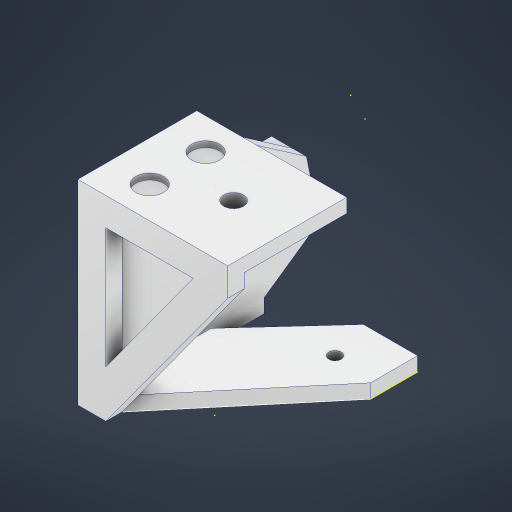
# Autodesk Inventor part: DC23[R][F][T1]
Saved by Autodesk Inventor 2024 (Build 280153000, 153)
## iProperties
Created: 2022-10-25
Part Number: DC23[R][F][T1]
Material: Aluminio 6061
Document SubType Name: Modeling
Designer: juanr
Density: 2.7 g/cm^3
Appearance: Aluminio - Plano
Mass: 248.976 g
Surface Area: 332.545 cm^2
Volume: 92.2132 cm^3
Author: juanr
Autodesk Inventor part; units mm, degrees
ref_plane "YZ Plane" through (0, 0, 0) normal (1, 0, 0) x (0, 1, 0)
ref_plane "XZ Plane" through (0, 0, 0) normal (0, 1, 0) x (-1, 0, 0)
ref_plane "XY Plane" through (0, 0, 0) normal (0, 0, 1) x (1, 0, 0)
sketch "Sketch1" plane through (0, 0, 0) normal (0, 1, 0) x (-1, 0, 0)
  line L0 (0, -25.5) -> (-34.15, -25.5)
  line L1 (-34.15, -25.5) -> (-34.15, 0)
  line L2 (-34.15, 0) -> (-34.15, 25.5)
  line L3 (-34.15, 25.5) -> (0, 25.5)
  line L4 (0, 25.5) -> (34.15, 25.5)
  line L5 (34.15, 25.5) -> (34.15, 0)
  line L6 (34.15, 0) -> (34.15, -25.5)
  line L7 (34.15, -25.5) -> (0, -25.5)
  point P0 (0, 0)
  constraints: 16 end point, 3 perpendicular, 2 point on line, 1 horizontal, 1 vertical
extrude "Extrusion1" add sketch "Sketch1" along normal blind 7
sketch "Sketch3" plane through (-34.15, 0, 25.5) normal (0, 0, 1) x (1, 0, 0)
  line L0 (0, 0) -> (0, -78.85)
  point P0 (34.15, 0)
  dimension "d7" = 78.85
  constraints: 2 end point, 1 vertical
  measures "d7" distance of L0.start L0.end
sketch "Sketch4" plane through (-34.15, 0, -25.5) normal (-1, 0, 0) x (0, 0, 1)
  line L0 (51, 0) -> (51, -78.85)
  line L1 (51, -78.85) -> (-39, -78.85)
  line L2 (-39, -78.85) -> (-39, -71.85)
  line L3 (0, 0) -> (-39, -71.85)
  line L4 (0, 0) -> (51, 0)
  point P0 (25.5, 0)
  dimension "d10" = 90
  dimension "d11" = 7
  constraints: 10 end point, 2 horizontal, 2 vertical
  measures "d10" distance of L0.end L1.end
  measures "d11" distance of L1.end L2.end
extrude "Extrusion2" add sketch "Sketch4" against normal blind 7
sketch "Sketch6" plane through (0, 7, 0) normal (0, 1, 0) x (1, 0, 0)
  line L0 (34.15, -25.5) -> (34.15, 25.5) projected
  line L1 (34.15, 25.5) -> (34.15, 0)
  line L2 (-34.15, 25.5) -> (-34.15, -25.5) projected
  circle A0 centre (8.15, 0) radius 5
  point P0 (0, 0)
  dimension "d20" = 10
  constraints: 2 end point, 1 centre point, 1 midpoint
  measures "d20" diameter of A0
extrude "Extrusion4" cut sketch "Sketch6" against normal blind 10
sketch "Sketch7" plane through (-27.15, 0, -25.5) normal (1, 0, 0) x (0, 0, -1)
  line L0 (-51, -78.85) -> (39, -78.85) projected
  line L1 (-51, -78.85) -> (39, -78.85)
  line L2 (39, -78.85) -> (39, -71.85) projected
  line L3 (39, -78.85) -> (39, -71.85)
  line L4 (39, -71.85) -> (-51, -71.85)
  line L5 (-51, 0) -> (-51, -78.85) projected
  line L6 (-51, -78.85) -> (-51, -71.85)
  point P0 (-25.5, 0)
  constraints: 8 end point, 2 perpendicular, 1 collinear, 1 horizontal, 1 point on line
sketch "Sketch8" plane through (0, 0, 0) normal (0, -1, 0) x (1, 0, 0)
  circle A0 centre (8.15, 0) radius 5 projected
  line L0 (8.15, 18.5) -> (34.15, 18.5)
  line L1 (34.15, 25.5) -> (34.15, -25.5) projected
  line L2 (8.15, 25.5) -> (34.15, 25.5)
  line L3 (8.15, 25.5) -> (-27.15, 25.5)
  line L4 (-27.15, 25.5) -> (-27.15, -25.5) projected
  line L5 (8.15, 18.5) -> (-27.15, 18.5)
  line L6 (34.15, 25.5) -> (34.15, 18.5)
  line L7 (-27.15, 25.5) -> (-27.15, 18.5)
  point P0 (0, 0)
  constraints: 12 end point, 2 collinear, 2 point on line, 1 horizontal, 1 parallel
extrude "Extrusion6" add sketch "Sketch7" along normal blind 58.5
extrude "Extrusion7" add sketch "Sketch8" along normal blind 78.75 contours L5 L4 L3 L2 L1 L0
sketch "Sketch9" plane through (31.35, 0, -25.5) normal (1, 0, 0) x (0, 0, -1)
  line L0 (-51, -78.75) -> (-51, 7) projected
  line L1 (-44, 0) -> (-44, -71.85) projected
  line L2 (-51, -78.75) -> (-44, -78.75)
  line L3 (-44, -78.75) -> (-44, -71.85)
  line L4 (-44, -71.85) -> (-51, -71.85)
  line L5 (-51, -71.85) -> (-51, -78.75)
  point P0 (-25.5, 0)
  constraints: 8 end point, 2 parallel, 1 horizontal, 1 perpendicular
extrude "Extrusion8" cut sketch "Sketch9" along normal blind 10
sketch "Sketch10" plane through (0, 7, 0) normal (0, 1, 0) x (1, 0, 0)
  point P0 (0, 0)
sketch "Boceto11" plane through (-34.15, -78.85, -64.5) normal (0, -1, 0) x (1, 0, 0)
  line L0 (72.0718, 89.9914) -> (72.0718, 37.9883)
  line L1 (72.0718, 37.9883) -> (65.5278, 37.9883)
  line L2 (65.5278, 37.9883) -> (65.5278, 89.9914)
  line L3 (72.0718, 89.9914) -> (72.0718, 92.1751)
  line L4 (72.0718, 92.1751) -> (65.5278, 92.1751)
  line L5 (65.5278, 92.1751) -> (65.5278, 89.9914)
  point P0 (34.15, 64.5)
  constraints: 12 end point, 2 perpendicular, 1 parallel, 1 vertical
extrude "Extrusión9" cut sketch "Boceto11" against normal blind 1000
sketch "Boceto18" plane through (-34.15, -78.85, 25.5) normal (0, 0, 1) x (1, 0, 0)
  point P0 (34.15, 78.85)
sketch "Boceto23" plane through (-27.15, 0, -25.5) normal (0, 0.4770514, -0.8788754) x (-1, 0, 0)
  point P0 (-27.15, 12.1648)
sketch "Boceto24" plane through (-27.15, 0, -25.5) normal (0, 0, -1) x (-1, 0, 0)
  line L0 (7, -71.85) -> (7, -78.85) projected
  line L1 (7, -78.35) -> (7, -78.85)
  line L2 (7, -78.85) -> (-58.5, -78.85) projected
  line L3 (-58.5, -78.85) -> (-58.5, -77.85)
  line L4 (-58.5, -71.85) -> (-58.5, -78.85) projected
  line L5 (-58.5, -77.85) -> (6, -77.85)
  line L6 (7, -77.85) -> (7, -78.85)
  line L7 (7, -78.85) -> (-58.8392, -78.85)
  line L8 (-58.5278, 7) -> (7, 7) projected
  line L9 (7, -78.85) -> (7, 7)
  line L10 (7, 7) -> (6, 7)
  line L11 (6, 6) -> (6, -77.85)
  line L12 (-58.5278, -71.85) -> (-58.5278, 7) projected
  line L13 (-58.5278, 7) -> (-58.5278, 6)
  line L14 (-58.5278, 6) -> (6, 6)
  line L15 (7, 0) -> (7, 7) projected
  line L16 (7, 6) -> (7, 7)
  line L17 (7, 7) -> (-58.5278, 7)
  point P0 (-27.15, 0)
  dimension "d65" = 1
  dimension "d66" = 1
  dimension "d67" = 1
  constraints: 24 end point, 7 perpendicular, 5 point on line, 1 collinear, 1 horizontal, 1 vertical
  measures "d65" distance of L2.end L3.end
  measures "d66" distance of L8.end L10.end
  measures "d67" distance of L8.start L13.end
extrude "Extrusión19" cut sketch "Boceto24" along normal mid plane 1000
sketch "Boceto25" plane through (31.35, -71.85, -64.5) normal (0, 0, -1) x (-1, 0, 0)
  point P0 (31.35, 71.85)
sketch "Boceto27" plane through (31.3778, 0, -25.5) normal (0, 0, -1) x (-1, 0, 0)
  line L0 (0, -71.85) -> (0, 6) projected
  line L1 (0, 6) -> (0.228, 6)
  line L2 (0, 6) -> (64.5278, 6) projected
  line L3 (0.228, 6) -> (0.228, -77.85)
  line L4 (0.0278, -77.85) -> (64.5278, -77.85) projected
  line L5 (0.0278, -71.85) -> (0.0278, -77.85) projected
  line L6 (0.228, -77.85) -> (0.0278, -77.85)
  line L7 (0.0278, -77.85) -> (0, 6)
  line L8 (0, 6) -> (0, -77.85)
  line L9 (0, -77.85) -> (0.0278, -77.85)
  point P0 (31.3778, 0)
  dimension "d73" = 0.228
  constraints: 12 end point, 3 perpendicular, 3 point on line, 1 horizontal
  measures "d73" distance of L0.end L1.end
extrude "Extrusión21" cut sketch "Boceto27" along normal mid plane 1000
sketch "Boceto28" plane through (-33.15, 0, -25.5) normal (-1, 0, 0) x (0, 0, 1)
  point P0 (25.5, 0)
sketch "Boceto30" plane through (-33.15, 0, -25.5) normal (-1, 0, 0) x (0, 0, 1)
  point P0 (25.5, 0)
sketch "Boceto31" plane through (-33.15, 0, -25.5) normal (-1, 0, 0) x (0, 0, 1)
  circle A0 centre (64.38, -38.5153) radius 2.6
  point P0 (25.5, 0)
  point P1 (64.38, -49.4573)
  constraints: 1 centre point
sketch "Boceto32" plane through (-27.15, -71.85, 18.5) normal (0, 1, 0) x (1, 0, 0)
  circle A0 centre (47, 71.5) radius 5 projected
  circle A1 centre (47, 71.5) radius 5
  line L0 (52, 71.5) -> (58.2998, 71.5)
  line L1 (67, 83) -> (67, -7)
  line L2 (58.2998, -7) -> (-6, -7) projected
  line L3 (67, -7) -> (58.2998, -7)
  line L4 (58.2998, -7) -> (58.2998, 83)
  line L5 (47, 76.5) -> (47, 83)
  line L6 (-6, 83) -> (0, 83) projected
  line L7 (-6, 83) -> (-6, 91.5)
  line L8 (-6, 91.5) -> (67, 91.5)
  line L9 (67, 91.5) -> (67, 83)
  line L10 (-6, 83) -> (58.2998, 83)
  point P0 (27.15, 18.5)
  constraints: 18 end point, 2 perpendicular, 2 point on circle, 2 point on line, 2 vertical, 1 centre point, 1 coincident, 1 collinear, 1 horizontal
extrude "Extrusión23" add sketch "Boceto32" against normal blind 6 contours L4 L10 L6 L7 L8 L9 L1 L3
sketch "Boceto33" plane through (-33.15, -77.85, 25.5) normal (-1, 0, 0) x (0, 0, 1)
  line L0 (0, 83.85) -> (0, 0) projected
  line L1 (0, 74.4354) -> (10.1255, 74.4354)
  line L2 (10.1255, 74.4354) -> (10.1255, 56.6115)
  line L3 (10.9445, 54.9975) -> (18.0243, 49.8171)
  line L4 (18.8039, 48.5979) -> (20.1084, 42.1205)
  line L5 (0, 11.6181) -> (18.1478, 11.6181)
  line L6 (20.1478, 13.6181) -> (20.1478, 41.7256)
  arc A0 (10.1255, 56.6115) -> (10.9445, 54.9975) centre (12.1255, 56.6115) ccw
  arc A1 (18.8039, 48.5979) -> (18.0243, 49.8171) centre (16.8433, 48.203) ccw
  arc A2 (20.1478, 41.7256) -> (20.1084, 42.1205) centre (18.1478, 41.7256) ccw
  arc A3 (18.1478, 11.6181) -> (20.1478, 13.6181) centre (18.1478, 13.6181) ccw
  point P0 (-25.5, 77.85)
  dimension "d91" = 2
  constraints: 12 end point, 8 point on circle, 8 tangent, 4 centre point, 3 equal radius, 2 horizontal, 2 perpendicular, 2 point on line
  measures "d91" radius of A0
extrude "Extrusión24" add sketch "Boceto33" against normal blind 6
extrude "Extrusión25" cut sketch "Boceto31" against normal blind 6
sketch "Boceto34" plane through (-27.15, -77.85, 25.5) normal (1, 0, 0) x (0, 0, -1)
  line L0 (-18.1478, 11.6181) -> (-21.8775, 11.6181)
  line L1 (-21.8775, 11.6181) -> (-21.8775, 48.067)
  line L2 (-21.8775, 48.067) -> (-10.1255, 56.8358)
  line L3 (-10.1255, 74.4354) -> (-10.1255, 56.6115) projected
  line L4 (-10.1255, 56.8358) -> (-10.1255, 48.9642)
  line L5 (-10.1255, 48.9642) -> (-16.6729, 42.1735)
  line L6 (-16.6729, 42.1735) -> (-18.1478, 11.6181)
  point P0 (25.5, 77.85)
  constraints: 12 end point, 1 horizontal, 1 perpendicular, 1 point on line, 1 vertical
extrude "Extrusión26" add sketch "Boceto34" against normal blind 6
fillet "Empalme5" radius 10 3 edges at (-30.15, -21.0142, 35.6255) (-30.15, -29.783, 47.3775) (-30.15, -66.2319, 47.3775)
sketch "Boceto37" plane through (-33.15, 6, 25.5) normal (0, 1, 0) x (1, 0, 0)
  circle A0 centre (41.3, 25.5) radius 6 projected
  line L0 (41.3, 25.5) -> (17.3, 25.5)
  line L1 (17.3, 25.5) -> (17.3, 13.5)
  line L2 (17.3, 13.5) -> (17.3, 37.5)
  circle A1 centre (17.3, 13.5) radius 6
  circle A2 centre (17.3, 37.5) radius 6
  point P0 (33.15, 25.5)
  dimension "d106" = 24
  dimension "d107" = 12
  dimension "d108" = 24
  dimension "d109" = 12
  dimension "d110" = 12
  constraints: 6 end point, 2 centre point, 2 coincident, 1 horizontal, 1 perpendicular, 1 point on line
  measures "d106" distance of L0.start L0.end
  measures "d107" distance of L0.end L1.end
  measures "d108" distance of L1.end L2.end
  measures "d109" diameter of A1
  measures "d110" diameter of A2
extrude "Extrusión29" cut sketch "Boceto37" against normal blind 2.5 contours A1 | A2
sketch "Boceto39" plane through (-27.15, -71.85, 18.5) normal (0, 1, 0) x (1, 0, 0)
  line L0 (58.2998, -7) -> (58.2998, 0)
  line L1 (58.2998, 44) -> (58.2998, 91.5)
  line L2 (-6, 91.5) -> (67, 91.5) projected
  line L3 (0, 0) -> (58.2998, 0) projected
  line L4 (58.2998, 0) -> (58.2998, -7) projected
  line L5 (58.2998, -7) -> (67, -7) projected
  line L6 (58.2998, -7) -> (67, -7)
  line L7 (67, 91.5) -> (-6, 91.5) projected
  line L8 (67, -7) -> (67, 91.5)
  line L9 (67, 91.5) -> (58.2998, 91.5)
  line L10 (58.2998, 0) -> (58.2998, 44)
  point P0 (27.15, 18.5)
  constraints: 12 end point, 3 collinear, 2 point on line, 1 perpendicular, 1 vertical
extrude "Extrusión31" cut sketch "Boceto39" against normal blind 10
sketch "Boceto41" plane through (-27.15, -71.85, 18.5) normal (0, 1, 0) x (1, 0, 0)
  line L0 (58.2998, 91.5) -> (58.2998, -7) projected
  line L1 (58.2998, 91.5) -> (31.7998, 91.5)
  line L2 (31.7998, 91.5) -> (31.7998, 65)
  line L3 (31.7998, 65) -> (58.2998, 65)
  line L4 (58.2998, 65) -> (58.2998, 91.5)
  circle A0 centre (31.7998, 65) radius 6
  point P0 (27.15, 18.5)
  dimension "d124" = 26.5
  dimension "d125" = 26.5
  dimension "d126" = 12
  constraints: 8 end point, 2 parallel, 1 centre point, 1 coincident, 1 horizontal, 1 perpendicular
  measures "d124" distance of L3.end L2.end
  measures "d125" distance of L2.end L1.end
  measures "d126" diameter of A0
extrude "Extrusión32" cut sketch "Boceto41" against normal blind 10 contours A0 L2 L3 | L3 L2 A0
sketch "Sketch42" plane through (-27.15, -71.85, 18.5) normal (0, 1, 0) x (1, 0, 0)
  circle A0 centre (31.7998, 65) radius 6 projected
  line L0 (31.7998, 71) -> (31.7998, 65)
  circle A1 centre (31.7998, 65) radius 18
  line L1 (0, 0) -> (0, 83) projected
  line L2 (0, 83) -> (31.7998, 83)
  line L3 (58.2998, 91.5) -> (-6, 91.5) projected
  line L4 (49.7998, 65) -> (49.7998, 0)
  line L5 (58.2998, 0) -> (0, 0) projected
  line L6 (0, 0) -> (58.2998, 0) projected
  line L7 (49.7998, 0) -> (58.2998, 0)
  line L8 (58.2998, 91.5) -> (58.2998, -7) projected
  line L9 (58.2998, 0) -> (58.2998, 91.5)
  line L10 (0, 83) -> (0, 44) projected
  line L11 (0, 83) -> (-6, 83)
  line L12 (-6, 91.5) -> (-6, 83) projected
  line L13 (-6, 83) -> (-6, 91.5)
  line L14 (58.2998, 91.5) -> (58.2998, 0) projected
  line L15 (-6, 91.5) -> (58.2998, 91.5)
  point P0 (27.15, 18.5)
  point P1 (58.2998, -7)
  dimension "d129" = 36
  constraints: 16 end point, 3 vertical, 2 collinear, 2 point on circle, 1 centre point, 1 coincident, 1 horizontal, 1 parallel, 1 perpendicular, 1 point on line, 1 vertical alignment, 2 other
  measures "d129" diameter of A1
extrude "Extrusion33" cut sketch "Sketch42" against normal blind 10 contours A1 L2 L11 L12 L3 L8 L5 L4
sketch "Sketch43" plane through (-27.15, -71.85, 18.5) normal (0, 0, -1) x (-1, 0, 0)
  line L0 (6, -6) -> (-58.2998, -6) projected
  line L1 (0, 0) -> (-49.7998, 0) projected
  line L2 (-58.2998, -6) -> (-49.7998, -6)
  line L3 (-49.7998, -6) -> (-49.7998, 0)
  line L4 (-49.7998, 0) -> (-58.2998, 0)
  line L5 (-58.2998, 0) -> (-58.2998, -6)
  point P0 (-27.15, 71.85)
  constraints: 8 end point, 2 parallel, 1 horizontal, 1 perpendicular
extrude "Extrusion34" add sketch "Sketch43" along normal blind 20
fillet "Fillet7" radius 7 1 edges at (31.1498, -74.85, -1.5)
fillet "Fillet8" radius 2 1 edges at (22.6498, -74.85, -1.5)
sketch "Sketch44" plane through (-33.15, 0, -25.5) normal (-1, 0, 0) x (0, 0, 1)
  line L0 (68.8577, -26.7837) -> (65.1452, -24.0136) projected
  line L1 (61.1255, -3.4146) -> (51, -3.4146) projected
  line L2 (65.1452, -24.0136) -> (51, -24.0136)
  line L3 (51, -24.0136) -> (51, -3.4146)
  line L4 (51, -3.4146) -> (65.1452, -3.4146)
  line L5 (65.1452, -3.4146) -> (65.1452, -24.0136)
  point P0 (25.5, 0)
  constraints: 8 end point, 2 parallel, 1 horizontal, 1 perpendicular
extrude "Extrusion35" cut sketch "Sketch44" against normal blind 20
sketch "Sketch45" plane through (-33.15, 6, 25.5) normal (0, 1, 0) x (1, 0, 0)
  circle A0 centre (41.3, 25.5) radius 5 projected
  circle A1 centre (41.3, 25.5) radius 4.25
  circle A2 centre (41.3, 25.5) radius 5
  point P0 (33.15, 25.5)
  dimension "d138" = 8.5
  constraints: 2 centre point, 2 coincident, 1 concentric
  measures "d138" diameter of A1
extrude "Extrusion36" add sketch "Sketch45" against normal blind 6
sketch "Sketch46" plane through (-33.15, 0, -25.5) normal (-1, 0, 0) x (0, 0, 1)
  point P0 (25.5, 0)
sketch "Sketch47" plane through (-33.15, 0, -25.5) normal (-1, 0, 0) x (0, 0, 1)
  line L0 (-44.1201, -43.7798) -> (-41.0263, -28.4947)
  line L1 (-39, -71.85) -> (0, 0) projected
  line L2 (-41.0263, -28.4947) -> (0, 0)
  line L3 (0, 0) -> (-39, -71.85)
  line L4 (-44.1201, -43.7798) -> (-44.1201, -71.85)
  line L5 (-44.1201, -71.85) -> (-39, -71.85)
  point P0 (25.5, 0)
  constraints: 10 end point, 1 collinear, 1 perpendicular, 1 vertical
extrude "Extrusion37" add sketch "Sketch47" against normal blind 6
sketch "Sketch48" plane through (-33.15, 6, -25.5) normal (-1, 0, 0) x (0, 0, 1)
  point P0 (25.5, -6)
sketch "Sketch49" plane through (-33.15, 6, -25.5) normal (-1, 0, 0) x (0, 0, 1)
  point P0 (25.5, -6)
sketch "Sketch50" plane through (-33.15, 6, -25.5) normal (-1, 0, 0) x (0, 0, 1)
  line L0 (-44.1201, -49.7798) -> (-41.0263, -34.4947) projected
  line L1 (-41.0263, -34.4947) -> (-46.4891, -61.4839)
  line L2 (-39, -83.85) -> (51, -83.85) projected
  line L3 (-39, -83.85) -> (-46.4891, -83.85)
  line L4 (-46.4891, -83.85) -> (-46.4891, -61.4839)
  line L5 (-41.0263, -34.4947) -> (-39, -69.2782)
  line L6 (-39, -69.2782) -> (-39, -83.85)
  point P0 (25.5, -6)
  constraints: 10 end point, 1 collinear, 1 horizontal, 1 perpendicular, 1 vertical
extrude "Extrusion38" add sketch "Sketch50" against normal blind 6
sketch "Sketch51" plane through (-33.15, 6, -25.5) normal (-1, 0, 0) x (0, 0, 1)
  line L0 (-41.0263, -34.4947) -> (-46.4891, -61.4839) projected
  line L1 (-41.0263, -34.4947) -> (-46.4891, -61.4839)
  line L2 (-46.4891, -61.4839) -> (-15.8808, -61.4839)
  line L3 (-41.0263, -34.4947) -> (-15.8808, -34.4947)
  line L4 (-15.8808, -34.4947) -> (-15.8808, -61.4839)
  point P0 (25.5, -6)
  constraints: 8 end point, 2 horizontal, 1 collinear, 1 perpendicular
extrude "Extrusion39" add sketch "Sketch51" along normal blind 9
sketch "Sketch52" plane through (-33.15, -55.4839, -71.9891) normal (0, -1, 0) x (1, 0, 0)
  line L0 (-9, 30.6084) -> (0, 53.8004)
  line L1 (0, 0) -> (0, 97.4891) projected
  line L2 (0, 30.6084) -> (0, 53.8004)
  line L3 (0, 30.6084) -> (-9, 30.6084)
  point P0 (33.15, 71.9891)
  constraints: 6 end point, 2 point on line, 1 collinear, 1 perpendicular
extrude "Extrusion40" add sketch "Sketch52" against normal blind 26.989
sketch "Sketch53" plane through (-33.15, -55.4839, -18.1887) normal (-0.9322642, 0, 0.3617781) x (0.3617781, 0, 0.9322642)
  point P0 (28.9496, 55.4839)
sketch "Sketch54" plane through (-33.15, 6, -25.5) normal (-1, 0, 0) x (0, 0, 1)
  line L0 (51, -72.2319) -> (51, -83.85) projected
  line L1 (51, -83.85) -> (86.3988, -83.85)
  line L2 (86.3988, -83.85) -> (86.3988, -18.2813)
  line L3 (86.3988, -18.2813) -> (51, -18.2813)
  line L4 (51, -18.2813) -> (51, -83.85)
  point P0 (25.5, -6)
  constraints: 8 end point, 2 parallel, 1 horizontal, 1 perpendicular
extrude "Extrusion41" cut sketch "Sketch54" against normal blind 26.989
sketch "Sketch55" plane through (-33.15, -55.4839, -71.9891) normal (0, 0.198384, -0.9801244) x (-1, 0, 0)
  line L0 (9, 6.0722) -> (9, 32.5248) projected
  line L1 (9, 17.5562) -> (3.5, 17.5562)
  line L2 (9, 17.5562) -> (14.5, 17.5562) construction
  circle A0 centre (3.5, 17.5562) radius 2.55
  point P0 (-33.15, 68.6627)
  dimension "d153" = 5.5
  dimension "d154" = 180
  dimension "d155" = 5.1
  constraints: 4 end point, 1 centre point, 1 coincident, 1 collinear, 1 horizontal, 1 perpendicular, 1 point on line
  measures "d153" distance of L1.start L1.end
  measures "d154" angle of L1 L2
  measures "d155" diameter of A0
extrude "Extrusion42" cut sketch "Sketch55" against normal blind 20
sketch "Sketch56" plane through (-33.15, -77.85, 25.5) normal (0, 0, 1) x (1, 0, 0)
  line L0 (0, 77.85) -> (0, 83.85) projected
  line L1 (0, 83.85) -> (12, 83.85)
  line L2 (64.2998, 83.85) -> (0, 83.85) projected
  line L3 (12, 83.85) -> (12, 0)
  line L4 (6, 0) -> (37.7998, 0) projected
  line L5 (0, 83.85) -> (0, 0) projected
  line L6 (12, 0) -> (0, 0)
  line L7 (0, 0) -> (0, 83.85)
  line L8 (0, 83.85) -> (12, 83.85)
  line L9 (12, 83.85) -> (12, 0)
  line L10 (0, 83.85) -> (64.3, 83.85)
  line L11 (64.3, 83.85) -> (64.3, 71.85)
  line L12 (64.3, 71.85) -> (0, 71.85)
  line L13 (0, 71.85) -> (0, 83.85)
  line L14 (64.2998, 0) -> (64.2998, 83.85) projected
  line L15 (64.3, 71.85) -> (12, 0)
  line L16 (64.3, 71.85) -> (54.5981, 78.9121)
  line L17 (12, 0) -> (3.5198, 8.4904)
  line L18 (3.5198, 8.4904) -> (54.5981, 78.9121)
  line L19 (12, 0) -> (64.2998, 0)
  line L20 (64.3, 71.85) -> (64.2998, 0)
  point P0 (33.15, 77.85)
  point P1 (37.7998, 0)
  point P2 (64.2998, 71.8497)
  point P3 (12, 20.182)
  point P4 (49.4758, 71.85)
  point P5 (12, 71.85)
  dimension "d158" = 12
  dimension "d159" = 64.3
  dimension "d160" = 12
  dimension "d161" = 12
  dimension "d162" = 12
  constraints: 32 end point, 4 parallel, 4 perpendicular, 3 horizontal, 2 point on line
  measures "d158" distance of L0.end L1.end
  measures "d159" distance of L11.end L12.end
  measures "d160" distance of L10.end L11.end
  measures "d161" distance of L11.end L16.end
  measures "d162" distance of L3.end L17.end
extrude "Extrusion43" cut sketch "Sketch56" against normal blind 20 contours L12 L18 L3 | L14 L19 L4 L15
sketch "Sketch57" plane through (-27.15, -77.85, -64.5) normal (0, -1, 0) x (1, 0, 0)
  point P0 (27.15, 64.5)
sketch "Sketch58" plane through (-27.15, -77.85, -64.5) normal (0, -1, 0) x (1, 0, 0)
  line L0 (0.0098, 82.9715) -> (6.0098, 82.9715)
  line L1 (0.0098, 82.9715) -> (58.6458, 82.9715)
  line L2 (58.6458, 82.9715) -> (58.6458, -19.949)
  line L3 (58.6458, -19.949) -> (0.0098, -19.949)
  line L4 (0.0098, -19.949) -> (0.0098, 82.9715)
  line L5 (58.6458, 1.7715) -> (22.1928, 1.7715)
  line L6 (22.1928, 1.7715) -> (0.0098, 16.0551)
  line L7 (0.0098, 16.0551) -> (0.0098, 82.9715)
  line L8 (58.6458, 1.7715) -> (58.6458, 39.0076)
  line L9 (58.6458, 1.7715) -> (22.1928, 1.7715)
  line L10 (58.6458, 38.2245) -> (58.6458, 1.7715)
  line L11 (58.6458, 38.2245) -> (6.0098, 82.9715)
  point P0 (15.0563, 101.6492)
  constraints: 24 end point, 3 point on line
extrude "Extrusion44" add sketch "Sketch58" against normal blind 6
extrude "Extrusion45" cut sketch "Sketch58" against normal blind 6
extrude "Extrusion46" add sketch "Sketch58" against normal blind 6 contours L0 L11 L2 L5 L6 L4
sketch "Sketch59" plane through (-27.15, 0, -25.5) normal (1, 0, 0) x (0, 0, -1)
  line L0 (46.4891, -77.85) -> (46.4891, -55.4839) projected
  line L1 (22.9449, -71.85) -> (22.9449, -77.85) projected
  line L2 (46.4891, -55.4839) -> (22.9449, -71.85)
  line L3 (22.9449, -71.85) -> (22.9449, -77.85)
  line L4 (22.9449, -77.85) -> (46.4891, -77.85)
  line L5 (46.4891, -55.4839) -> (46.4891, -77.85) projected
  line L6 (46.4891, -77.85) -> (46.4891, -55.4839)
  line L7 (46.4891, -55.4839) -> (46.4891, -77.85)
  point P0 (-25.5, 0)
  constraints: 10 end point, 2 perpendicular, 1 collinear, 1 vertical
extrude "Extrusion47" cut sketch "Sketch59" along normal blind 0.1 and the other way blind 6
sketch "Sketch60" plane through (-4.9572, -77.85, -62.7285) normal (0, -1, 0) x (1, 0, 0)
  line L0 (36.107, 88.2285) -> (-22.1928, 88.2285) projected
  line L1 (36.107, 88.2285) -> (14.607, 88.2285)
  line L2 (14.607, 88.2285) -> (14.607, 20.7285)
  line L3 (14.607, 20.7285) -> (36.107, 20.7285)
  line L4 (36.107, 20.7285) -> (36.107, 88.2285)
  circle A0 centre (14.607, 20.7285) radius 2.7
  point P0 (4.9572, 62.7285)
  dimension "d176" = 21.5
  dimension "d177" = 67.5
  dimension "d178" = 5.4
  constraints: 8 end point, 2 parallel, 1 centre point, 1 coincident, 1 horizontal, 1 perpendicular
  measures "d176" distance of L3.end L2.end
  measures "d177" distance of L2.end L1.end
  measures "d178" diameter of A0
extrude "Extrusion48" cut sketch "Sketch60" against normal blind 10 contours A0 L3 L2 | L2 L3 A0
sketch "Sketch61" plane through (-33.15, -77.85, 25.5) normal (0, -1, 0) x (1, 0, 0)
  line L0 (64.6458, -51.7755) -> (64.6458, -88.2285) projected
  line L1 (64.6458, -88.2285) -> (64.6458, -70.002)
  line L2 (12, -7) -> (49.4758, -7) projected
  line L3 (64.6458, -70.002) -> (12, -7)
  line L4 (12, -7) -> (64.6458, -48.437)
  line L5 (64.6458, -48.437) -> (64.6458, -70.002)
  line L6 (64.6458, -88.2285) -> (46.4193, -88.2285)
  line L7 (6.1, -74.0029) -> (28.1928, -88.2285) projected
  line L8 (46.4193, -88.2285) -> (28.1928, -88.2285)
  line L9 (28.1928, -88.2285) -> (6.1, -61.7897)
  line L10 (6.1, -61.7897) -> (6.1, -74.0029)
  line L11 (6.1, -74.0029) -> (28.1928, -88.2285)
  point P0 (33.15, -25.5)
  dimension "d181" = 18.2265
  dimension "d182" = 18.2265
  constraints: 18 end point, 3 collinear, 1 horizontal, 1 midpoint, 1 parallel, 1 perpendicular, 1 point on line
  measures "d181" distance of L0.end L1.end
  measures "d182" distance of L0.end L6.end
extrude "Extrusion49" cut sketch "Sketch61" against normal blind 6
sketch "Sketch62" plane through (-33.15, -28.4947, -66.5263) normal (0, 0.198384, -0.9801244) x (-1, 0, 0)
  point P0 (-33.15, 41.1261)
sketch "Sketch63" plane through (-33.15, -77.85, 25.5) normal (0, -1, 0) x (1, 0, 0)
  line L0 (6, -7) -> (6, -51) projected
  line L1 (6, -7) -> (12, -7) projected
  line L2 (12, -7) -> (64.6458, -70.002)
  circle A0 centre (42.7998, -67.5) radius 2.7 projected
  line L3 (64.6458, -70.002) -> (42.7998, -67.5)
  line L4 (42.7998, -67.5) -> (53.7228, -80.5717)
  line L5 (53.7228, -80.5717) -> (64.6458, -70.002)
  line L6 (53.7228, -80.5717) -> (42.7996, -91.1416)
  line L7 (42.7996, -91.1416) -> (6, -51)
  line L8 (42.7996, -91.1416) -> (64.6458, -91.1416)
  line L9 (64.6458, -91.1416) -> (64.6458, -70.002)
  line L10 (6, -7) -> (73.4518, -7)
  line L11 (73.4518, -7) -> (73.4518, -117.9576)
  line L12 (73.4518, -117.9576) -> (6, -117.9576)
  line L13 (6, -117.9576) -> (6, -7)
  point P0 (33.15, -25.5)
  constraints: 24 end point, 3 parallel, 2 horizontal, 2 perpendicular, 1 point on line
extrude "Extrusion50" cut sketch "Sketch63" against normal blind 6 contours L7 L8 L9 L2 L10 L11 L12 L13
extrude "Extrusion51" add sketch "Sketch63" against normal blind 6 contours L1 L2 L3 A0 L4 L6 L7 L0 | L6 L5 L9 L8 | L5 L4 A0 L3
sketch "Sketch64" plane through (-33.15, -77.85, 25.5) normal (0, -1, 0) x (1, 0, 0)
  circle A0 centre (42.7998, -67.5) radius 2.7 projected
  line L0 (42.7998, -67.5) -> (42.7998, -70.2)
  line L1 (42.7998, -70.2) -> (42.7998, -85.2)
  line L2 (12, -7) -> (49.4758, -7) projected
  line L3 (12, -7) -> (64.6458, -70.002) projected
  line L4 (12, -7) -> (64.6458, -70.002)
  line L5 (64.6458, -70.002) -> (64.6458, -91.1416) projected
  line L6 (64.6458, -70.002) -> (64.6458, -91.1416)
  line L7 (64.6458, -91.1416) -> (42.7998, -91.1416)
  line L8 (6, -7) -> (6, -51) projected
  line L9 (42.7998, -91.1416) -> (6, -51)
  line L10 (42.7998, -85.2) -> (64.6458, -85.2)
  line L11 (45.4998, -67.5) -> (60.4998, -67.5)
  line L12 (60.4998, -67.5) -> (60.4998, -85.2)
  line L13 (60.4998, -67.5) -> (60.4998, -65.0404)
  line L14 (42.7998, -85.2) -> (37.3528, -85.2)
  line L15 (37.3528, -85.2) -> (67.2046, -85.2)
  line L16 (67.2046, -85.2) -> (67.2046, -95.398)
  line L17 (67.2046, -95.398) -> (37.3528, -95.398)
  line L18 (37.3528, -95.398) -> (37.3528, -85.2)
  line L19 (60.4998, -85.2) -> (70.2528, -85.2)
  line L20 (70.2528, -85.2) -> (70.2528, -62.331)
  line L21 (70.2528, -62.331) -> (60.4998, -62.331)
  line L22 (60.4998, -62.331) -> (60.4998, -85.2)
  point P0 (33.15, -25.5)
  dimension "d192" = 15
  dimension "d193" = 15
  constraints: 38 end point, 6 equal length, 5 perpendicular, 5 point on line, 4 horizontal, 2 point on circle, 2 vertical
  measures "d192" distance of L0.end L1.end
  measures "d193" distance of L11.start L11.end
extrude "Extrusion52" cut sketch "Sketch64" against normal blind 6 contours L13 L3 L5 L10 L12 | L10 L5 L7 L9 L14 | L22 L21 L20 L19 L15 L5 L3 | L9 L7 L5 L15 L16 L17 L18
sketch "Sketch65" plane through (-33.15, -77.85, 25.5) normal (0, -1, 0) x (1, 0, 0)
  line L0 (12, -7) -> (60.4998, -65.0404) projected
  line L1 (60.4998, -65.0404) -> (48.9264, -75.1202)
  line L2 (60.4998, -65.0404) -> (60.4998, -85.2) projected
  line L3 (60.4998, -65.0404) -> (60.4998, -85.2)
  line L4 (48.9264, -75.1202) -> (60.4998, -88.4085)
  line L5 (60.4998, -65.0404) -> (58.8524, -86.517)
  line L6 (58.8524, -86.517) -> (37.3528, -85.2002)
  line L7 (37.3528, -85.2002) -> (48.9264, -75.1202)
  line L8 (58.8524, -86.517) -> (69.5954, -86.517)
  line L9 (69.5954, -86.517) -> (69.5954, -59.5334)
  line L10 (69.5954, -59.5334) -> (58.8524, -59.5334)
  line L11 (58.8524, -59.5334) -> (58.8524, -86.517)
  point P0 (33.15, -25.5)
  point P1 (58.8524, -63.069)
  dimension "d196" = 15.3475
  constraints: 20 end point, 2 parallel, 1 horizontal, 1 perpendicular, 1 point on line, 1 vertical
  measures "d196" distance of L0.end L1.end
extrude "Extrusion53" cut sketch "Sketch65" against normal blind 6 contours L11 L10 L9 L8 L5 L0
extrude "Extrusion54" add sketch "Sketch65" against normal blind 6 contours L5 L11 L1 | L11 L4 L1 | L6 L7 L4
sketch "Sketch66" plane through (-33.15, -77.85, 25.5) normal (0, -1, 0) x (1, 0, 0)
  line L0 (37.3528, -85.2) -> (60.4998, -85.2)
  line L1 (60.4998, -85.2) -> (60.4998, -65.0404)
  line L2 (60.4998, -65.0404) -> (37.3528, -65.0404)
  line L3 (37.3528, -65.0404) -> (37.3528, -85.2)
  line L4 (74.8766, -52.5753) -> (26.3032, -52.5753)
  line L5 (26.3032, -52.5753) -> (26.3032, -106.4614)
  line L6 (26.3032, -106.4614) -> (74.8766, -106.4614)
  line L7 (74.8766, -106.4614) -> (74.8766, -52.5753)
  line L8 (60.4998, -52.5753) -> (60.4998, -85.2)
  line L9 (26.3032, -85.2) -> (39.2055, -85.2)
  line L10 (60.4998, -65.0404) -> (39.2055, -85.2)
  point P0 (33.15, -25.5)
  constraints: 22 end point, 4 parallel, 4 point on line, 2 horizontal, 2 perpendicular, 1 vertical
extrude "Extrusion55" cut sketch "Sketch66" against normal blind 6 contours L0 L1 L8 L4 L7 L6 L5 L9
extrude "Extrusion56" add sketch "Sketch66" against normal blind 6 contours L10 L1 L0
sketch "Sketch67" plane through (-33.15, -77.85, 25.5) normal (0, -1, 0) x (1, 0, 0)
  point P0 (33.15, -25.5)
sketch "Sketch68" plane through (-33.15, -77.85, 25.5) normal (0, -1, 0) x (1, 0, 0)
  line L0 (60.4998, -65.0404) -> (60.4998, -85.2) projected
  line L1 (60.4998, -85.2) -> (37.3526, -85.2) projected
  line L2 (60.4998, -85.2) -> (37.3526, -85.2)
  line L3 (37.3526, -85.2) -> (6, -51)
  line L4 (6, -51) -> (6, -7)
  line L5 (6, -7) -> (12.2668, -7)
  line L6 (12, -7) -> (60.4998, -65.0404) projected
  line L7 (60.4998, -65.0404) -> (12, -7)
  circle A0 centre (42.7998, -67.5) radius 2.7 projected
  circle A1 centre (42.7998, -67.5) radius 2.7
  point P0 (33.15, -25.5)
  constraints: 10 end point, 2 collinear, 1 centre point, 1 coincident
body "Solid1"
